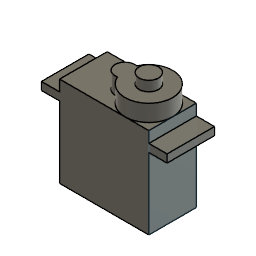
MG90S servo model (Autodesk Fusion 360 design; units mm, degrees)
part number: 2026-07-24-13-32-31-393
Autodesk Fusion 360 part; units mm, degrees
sketch "Sketch1" plane through (0, 0, 0) normal (0, 1, 0) x (1, 0, 0)
  line L0 (0, 0) -> (22.5, 0)
  line L1 (22.5, 0) -> (22.5, 12)
  line L2 (22.5, 12) -> (0, 12)
  line L3 (0, 12) -> (0, 0)
  dimension "d1" = 22.5
  dimension "d2" = 12
  constraint horizontal L0
  constraint vertical L1
  constraint horizontal L2
  constraint vertical L3
  constraint coincident L0.start L3.end
  measures "d1" distance of L0.start L0.end
  measures "d2" distance of L0.start L2.end
extrude "Extrude1" add sketch "Sketch1" along normal blind 22.8
sketch "Sketch2" plane through (22.5, 0, 0) normal (1, 0, 0) x (0, 0, -1)
  line L0 (0, 0) -> (12, 0)
  line L1 (12, 0) -> (12, 22.8)
  line L2 (12, 22.8) -> (0, 22.8)
  line L3 (0, 22.8) -> (0, 0)
sketch "Sketch3" plane through (0, 22.8, 0) normal (0, 1, 0) x (-1, 0, 0)
  line L0 (0, -12) -> (0, 0)
  line L1 (0, 0) -> (-22.5, 0)
  line L2 (-22.5, 0) -> (-22.5, -12)
  line L3 (-22.5, -12) -> (0, -12)
  line L4 (-22.5, -6) -> (-16.5, -6) construction
  circle A0 centre (-16.5, -6) radius 6
  line L5 (-16.5, -6) -> (0, -6) construction
  circle A1 centre (-10.5, -6) radius 2.5
  dimension "d5" = 6
  dimension "d6" = 12
  dimension "d16" = 5
  constraint midpoint L2 L4.start
  constraint perpendicular L2 L4
  constraint coincident L4.end A0.centre
  constraint midpoint L0 L5.end
  constraint coincident A0 A1.centre
  constraint coincident L5 A1.centre
  measures "d5" distance of L4.start L4.end
  measures "d6" diameter of A0
  measures "d16" diameter of A1
extrude "Extrude2" add sketch "Sketch3" along normal blind 4.2 contours A0 A1 | A0 A1 | A0 A1
sketch "Sketch4" plane through (0, 27, 0) normal (0, 1, 0) x (-1, 0, 0)
  arc A0 (-11.0208, -8.4451) -> (-11.0208, -3.5549) centre (-10.5, -6) ccw
  arc A1 (-11.0208, -3.5549) -> (-11.0208, -8.4451) centre (-16.5, -6) ccw
  circle A2 centre (-16.5, -6) radius 2.45
  dimension "d17" = 4.9
  constraint concentric A1 A2
  measures "d17" diameter of A2
sketch "Sketch5" plane through (22.5, 0, 0) normal (1, 0, 0) x (0, 0, -1)
  line L0 (12, 18) -> (0, 18)
  line L1 (0, 18) -> (0, 20)
  line L2 (0, 20) -> (12, 20)
  line L3 (12, 20) -> (12, 18)
  constraint horizontal L0
  constraint vertical L1
  constraint horizontal L2
  constraint vertical L3
extrude "Extrude4" add sketch "Sketch5" along normal blind 4.6
sketch "Sketch8" plane through (0, 0, 0) normal (-1, 0, 0) x (0, 0, 1)
  line L0 (-12, 0) -> (0, 0)
  line L1 (0, 0) -> (0, 22.8)
  line L2 (0, 22.8) -> (-12, 22.8)
  line L3 (-12, 22.8) -> (-12, 0)
  line L4 (-12, 20) -> (0, 20)
  line L5 (0, 20) -> (0, 18)
  line L6 (0, 18) -> (-12, 18)
  line L7 (-12, 18) -> (-12, 20)
extrude "Extrude5" add sketch "Sketch8" along normal blind 4.6 contours L1 L3 L4 L5 L6 L7
extrude "Extrude6" add sketch "Sketch4" along normal blind 2.5 contours A2
